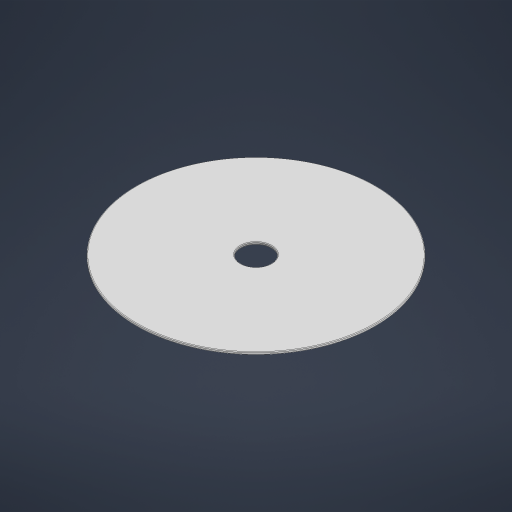
# Autodesk Inventor part: CD
Saved by Autodesk Inventor 2024.1 (Build 281209000, 209)
## iProperties
Created: 2024-11-17
Part Number: CD
Material: Generic
Document SubType Name: Modeling
Designer: Designer
Density: 1 g/cm^3
Appearance: Default
Author: Designer
Autodesk Inventor part; units mm, degrees
ref_plane "YZ Plane" through (0, 0, 0) normal (1, 0, 0) x (0, 1, 0)
ref_plane "XZ Plane" through (0, 0, 0) normal (0, 1, 0) x (-1, 0, 0)
ref_plane "XY Plane" through (0, 0, 0) normal (0, 0, 1) x (1, 0, 0)
sketch "Sketch1" plane through (0, 0, 0) normal (0, 1, 0) x (-1, 0, 0)
  circle A0 centre (0, 0) radius 7.62
  circle A1 centre (0, 0) radius 59.69
  dimension "d0" = 15.24
  dimension "d1" = 119.38
  constraints: 2 centre point, 2 coincident
  measures "d0" diameter of A0
  measures "d1" diameter of A1
extrude "Extrusion1" add sketch "Sketch1" along normal blind 1.27
fillet "Fillet1" radius 0.3175 4 edges at (59.69, 1.27, 0) (59.69, 0, 0) (7.62, 1.27, 0) (7.62, 0, 0)
body "Solid1"
